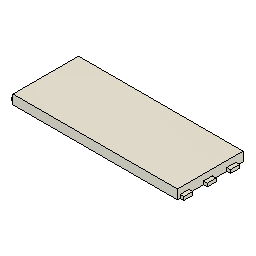
Parametric Centerpiece Template (Autodesk Fusion 360 design; units mm, degrees)
Autodesk Fusion 360 part; units mm, degrees
sketch "Base" plane through (0, 0, 0) normal (0, 1, 0) x (1, 0, 0) in component "DDD Wall Control Center Piece Parametric Template"
  line L0 (87.795, -35) -> (-87.795, -35)
  line L1 (-87.795, -35) -> (-87.795, 35)
  line L2 (-87.795, 35) -> (87.795, 35)
  line L3 (87.795, 35) -> (87.795, -35)
  line L4 (87.795, -35) -> (-87.795, 35) construction
  line L5 (-87.795, -35) -> (87.795, 35) construction
  dimension "d1" = 175.59
  dimension "d2" = 70
  constraint horizontal L0
  constraint perpendicular L0 L1
  constraint parallel L0 L2
  constraint parallel L1 L3
  constraint coincident L4 origin
  constraint coincident L5 origin
  constraint vertical L1
  measures "d1" distance of L1.end L2.end
  measures "d2" distance of L0.end L1.end
extrude "Extrude1" add sketch "Base" along normal blind 10 in component "DDD Wall Control Center Piece Parametric Template"
sketch "Mounting Tab" plane through (0, 0, 0) normal (1, 0, 0) x (0, 0, 1) in component "DDD Wall Control Center Piece Parametric Template"
  line L0 (-17.75, -3.5) -> (-27.25, -3.5)
  line L1 (-27.25, -3.5) -> (-27.25, 0)
  line L2 (-27.25, 0) -> (-17.75, 0)
  line L3 (-17.75, 0) -> (-17.75, -3.5)
  line L4 (-17.75, -3.5) -> (-27.25, 0) construction
  line L5 (-27.25, -3.5) -> (-17.75, 0) construction
  line L6 (1.75, 0) -> (22.5, 0)
  point P0 (-22.5, -1.75)
  dimension "d34" = 9.5
  dimension "d35" = 3.5
  dimension "d147" = 17.75
  constraint horizontal L0
  constraint perpendicular L0 L1
  constraint parallel L0 L2
  constraint parallel L1 L3
  constraint coincident L4 P0
  constraint coincident L5 P0
  constraint collinear L2 L6
  measures "d34" distance of L1.end L2.end
  measures "d35" distance of L0.end L1.end
  measures "d147" horizontal distance of L2.end origin
extrude "Extrude3" add sketch "Mounting Tab" along normal blind 4 from surface at 87.795 in component "DDD Wall Control Center Piece Parametric Template"
extrude "Extrude6" add sketch "Mounting Tab" against normal blind 4 from surface at -87.795 in component "DDD Wall Control Center Piece Parametric Template"
pattern_linear "R-Pattern3" count 1 spacing 0 along (0, -1, 0) count 3 spacing 25 along (0, 0, 1) of "Extrude3", "Extrude6" in component "DDD Wall Control Center Piece Parametric Template"
component "DDD Wall Control Center Piece Parametric Template" placed x (1, 0, 0) y (0, 1, 0) z (0, 0, 1) at (0, 0, 0)
equation "d1 = MMCenterPieceWidth"
equation "d2 = CenterPieceDepth"
equation "CenterPieceWidthUnits = 7" comment "Number of width spaces on the wall control pegboard.  Minimum 1,  maximum 14 for vertical wall control panels,  and 31 for horizonal panels.  Realistically your printer dimensions will determin how big you can make this."
equation "MMCenterPieceWidth = ( CenterPieceWidthUnits * 25.4 mm ) - 2.21 mm" comment "Don't change this.  Change CenterPieceWidthUnits instead.  Final width dimension subtracts 2.21mm from the standard 1\" space between wall control slots to account for the tabs for mouting into the slots"
equation "CenterPieceDepth = 70 mm" comment "Depth measurement from the wall control board extending out into space.  Minimum 17mm to fit at least one mounting tab.  Maximum  ¯\\_(ツ)_/¯"
equation "CenterPieceThickness = 2 mm" comment "Lower measurements make for good shelf-like objects,  taller measurement make for better custom tool holders"
equation "d147 = CenterPieceDepth / 2 - 17.25 mm"
equation "CountMountingTabs = 3" comment "Specify the number of mounting tabs to attach a sidepiece"
equation "d158 = CountMountingTabs"
equation "HowToUse = 0" comment "Insert this into a new design, and then break the link to the original to preserve the template.  Then modify as needed for centerpiece tool holders."
named bodies: "Center Piece Parametric Template"
